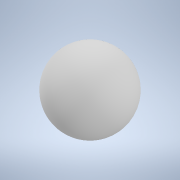
# Autodesk Inventor part: 76. Шарик фиксатора
Saved by Autodesk Inventor 2021 (Build 250183000, 183)
## iProperties
Created: 2021-04-09
Part Number: 76. Шарик фиксатора
Material: Типовые
Document SubType Name: Modeling
Designer: Данил
Density: 1 g/cm^3
Appearance: По умолчанию
Author: Данил
Autodesk Inventor part; units mm, degrees
ref_plane "YZ Plane" through (0, 0, 0) normal (1, 0, 0) x (0, 1, 0)
ref_plane "XZ Plane" through (0, 0, 0) normal (0, 1, 0) x (-1, 0, 0)
ref_plane "XY Plane" through (0, 0, 0) normal (0, 0, 1) x (1, 0, 0)
sketch "Эскиз1" plane through (0, 0, 0) normal (0, 0, 1) x (1, 0, 0)
  line L0 (0, 4.75) -> (0, -4.75)
  arc A0 (0, -4.75) -> (0, 4.75) centre (0, 0) ccw
  dimension "d0" = 4.75
  constraints: 2 coincident, 2 end point, 2 point on circle, 1 centre point, 1 midpoint, 1 vertical
  measures "d0" radius of A0
revolve "Вращение1" add sketch "Эскиз1" angle 360 about axis through (0, 4.75, 0) along (0, -1, 0)
